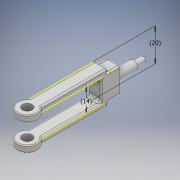
# Autodesk Inventor part: 앞바퀴스탠드
Saved by Autodesk Inventor 2018 (Build 220112000, 112)
## iProperties
Created: 2019-11-14
Part Number: 앞바퀴스탠드
Material: 일반
Document SubType Name: Modeling
Designer: LeeYounSeo
Density: 1 g/cm^3
Appearance: 기본값
Author: LeeYounSeo
Autodesk Inventor part; units mm, degrees
ref_plane "YZ Plane" through (0, 0, 0) normal (1, 0, 0) x (0, 1, 0)
ref_plane "XZ Plane" through (0, 0, 0) normal (0, 1, 0) x (-1, 0, 0)
ref_plane "XY Plane" through (0, 0, 0) normal (0, 0, 1) x (1, 0, 0)
sketch "스케치1" plane through (0, 0, 0) normal (0, 1, 0) x (-1, 0, 0)
  line L0 (0, 0) -> (8, 0)
  line L1 (8, 0) -> (8, -15)
  line L2 (8, -15) -> (0, -15)
  line L3 (0, -15) -> (0, 0)
  dimension "d0" = 15
  dimension "d1" = 8
  constraints: 8 end point, 2 parallel, 1 horizontal, 1 perpendicular
  measures "d0" distance of L0.end L1.end
  measures "d1" distance of L1.end L2.end
extrude "돌출1" add sketch "스케치1" along normal blind 8
sketch "스케치2" plane through (0, 8, 0) normal (0, 1, 0) x (1, 0, 0)
  circle A0 centre (-4, 7.5) radius 2.5
  line L0 (0, 15) -> (-8, 15) projected
  line L1 (0, 0) -> (0, 15) projected
  dimension "d4" = 5
  dimension "d5" = 7.5
  dimension "d6" = 4
  constraints: 1 centre point
  measures "d4" diameter of A0
  measures "d5" distance from line of L0 A0.centre
  measures "d6" distance from line of L1 A0.centre
extrude "돌출2" add sketch "스케치2" along normal blind 12
sketch "스케치3" plane through (-4, 20, -7.5) normal (0, 1, 0) x (1, 0, 0)
  circle A0 centre (0, 0) radius 1.5
  point P0 (4, -7.5)
  dimension "d9" = 3
  constraints: 1 centre point
  measures "d9" diameter of A0
extrude "돌출3" add sketch "스케치3" along normal blind 6
sketch "스케치4" plane through (0, 0, 0) normal (0, -1, 0) x (1, 0, 0)
  line L0 (-8, 2.5) -> (0, 2.5)
  line L1 (0, 2.5) -> (0, -17.5)
  line L2 (0, -17.5) -> (-8, -17.5)
  line L3 (-8, -17.5) -> (-8, 2.5)
  line L4 (0, -15) -> (0, 0) projected
  line L5 (-8, 0) -> (-8, -15) projected
  line L6 (0, 0) -> (-8, 0) projected
  line L7 (-8, -15) -> (0, -15) projected
  dimension "d12" = 2.5
  dimension "d13" = 2.5
  constraints: 8 end point, 2 collinear, 2 parallel, 1 horizontal, 1 perpendicular
  measures "d12" distance between parallel lines of L6 L0
  measures "d13" distance between parallel lines of L2 L7
extrude "돌출4" add sketch "스케치4" along normal blind 45
sketch "스케치5" plane through (0, 8, 0) normal (1, 0, 0) x (0, 0, -1)
  line L0 (1.5, -57) -> (13.5, -57)
  line L1 (13.5, -57) -> (13.5, -12)
  line L2 (13.5, -12) -> (1.5, -12)
  line L3 (1.5, -12) -> (1.5, -57)
  line L4 (-2.5, -8) -> (-2.5, -53) projected
  line L5 (17.5, -8) -> (17.5, -53) projected
  line L6 (0, 0) -> (15, 0) projected
  line L7 (17.5, -53) -> (-2.5, -53) projected
  point P0 (0, -8)
  dimension "d16" = 4
  dimension "d17" = 4
  dimension "d18" = 12
  dimension "d19" = 41
  dimension "d20" = 45
  constraints: 8 end point, 2 parallel, 1 horizontal, 1 perpendicular
  measures "d16" distance between parallel lines of L3 L4
  measures "d17" distance between parallel lines of L5 L1
  measures "d18" distance between parallel lines of L6 L2
  measures "d19" distance between parallel lines of L2 L7
  measures "d20" distance between parallel lines of L2 L0
sketch "스케치6" plane through (0, 8, 0) normal (1, 0, 0) x (0, 0, -1)
  point P0 (0, -8)
extrude "돌출5" cut sketch "스케치5" against normal blind 10
sketch "스케치7" plane through (-8, 0, 2.5) normal (0, 0, 1) x (1, 0, 0)
  line L0 (0, -45) -> (8, -45) projected
  circle A0 centre (4, -45) radius 6
  point P0 (8, 0)
  dimension "d23" = 12
  constraints: 1 centre point, 1 midpoint
  measures "d23" diameter of A0
extrude "돌출6" add sketch "스케치7" against normal blind 4
sketch "스케치8" plane through (-8, 0, 2.5) normal (0, 0, 1) x (1, 0, 0)
  circle A0 centre (4, -45) radius 2.95
  arc A1 (0, -40.5279) -> (8, -40.5279) centre (4, -45) ccw projected
  point P0 (8, 0)
  dimension "d26" = 5.9
  dimension "d27" = 0
  dimension "d28" = 0
  constraints: 1 centre point
  measures "d26" diameter of A0
  measures "d27" distance of A1.centre A0.centre
  measures "d28" distance of A1.centre A0.centre
extrude "돌출7" cut sketch "스케치8" against normal blind 4
sketch "스케치9" plane through (0, 0, -17.5) normal (0, 0, -1) x (-1, 0, 0)
  line L0 (8, -45) -> (0, -45) projected
  circle A0 centre (4, -45) radius 6
  circle A1 centre (4, -45) radius 2.95
  circle A2 centre (4, -45) radius 2.95 projected
  point P0 (0, 0)
  constraints: 2 centre point, 1 coincident, 1 midpoint
extrude "돌출8" add sketch "스케치9" against normal blind 4
sketch "스케치10" plane through (0, 0, -17.5) normal (0, 0, -1) x (-1, 0, 0)
  line L0 (1.05, -45) -> (6.95, -45) projected
  circle A0 centre (4, -45) radius 2.95
  point P0 (0, 0)
  constraints: 1 centre point, 1 midpoint
extrude "돌출9" cut sketch "스케치10" against normal blind 4
fillet "모깎기1" radius 1 26 edges at (-8, -20.2639, 2.5) (-4, 0, 2.5) (-8, 0, 1.25) (-4, 0, 0) (-8, 4, 0) (-4, 8, 0) (-8, 8, -7.5) (0, 8, -7.5) (0, 4, 0) (0, -20.2639, 2.5) (0, 0, 1.25) (-8, 4, -15) (-8, 0, -16.25) (-8, -20.2639, -17.5) (-8, -4, -7.5) (-8, -22.2639, -13.5) (0, -22.2639, -13.5) (-8, -22.2639, -1.5) (0, -20.2639, -17.5) (0, 0, -16.25) (0, 4, -15) (-4, 8, -15) (0, -4, -7.5) (0, -22.2639, -1.5) (-4, 0, -15) (-4, 0, -17.5)
fillet "모깎기2" radius 0.5 11 edges at (-6.5, 20, -7.5) (-5.5, 26, -7.5) (-6.5, 8, -7.5) (-7.5187, -40.1401, 2.5) (-0.4813, -40.1401, 2.5) (-7.5187, -40.1401, -1.5) (-0.4813, -40.1401, -1.5) (-0.4813, -40.1401, -13.5) (-7.5187, -40.1401, -13.5) (-0.4813, -40.1401, -17.5) (-7.5187, -40.1401, -17.5)
fillet "모깎기3" radius 2 6 edges at (-7.7071, -3.7071, -13.7929) (-0.2929, -3.7071, -13.7929) (-4, -4, -13.5) (-7.7071, -3.7071, -1.2071) (-0.2929, -3.7071, -1.2071) (-4, -4, -1.5)
sketch "스케치11" plane through (0, -40.5279, -16.5) normal (1, 0, 0) x (0, 0, -1)
  line L0 (-2, 0) -> (-2, 37.5279) projected
  line L1 (-16, 37.5279) -> (-16, 0) projected
  point P0 (-16.5, 40.5279)
  dimension "d38" = 14
  measures "d38" distance between parallel lines of L0 L1
sketch "스케치12" plane through (-8, -40.5279, 1.5) normal (-1, 0, 0) x (0, 0, 1)
  line L0 (1, 0.1376) -> (1, 39.5279) projected
  line L1 (-19, 39.5279) -> (-19, 0.1376) projected
  point P0 (-1.5, 40.5279)
  dimension "d39" = 20
  measures "d39" distance between parallel lines of L0 L1
